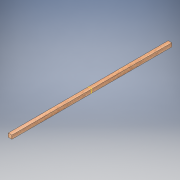
# Autodesk Inventor part: CAR_003_PoplarBrace
Saved by Autodesk Inventor 2018 (Build 220112000, 112)
## iProperties
Created: 2020-01-29
Part Number: CAR_003_PoplarBrace
Material: Wood (Birch)
Document SubType Name: Modeling
Designer: user
Mass: 41.2898 g
Surface Area: 240.193 cm^2
Volume: 75.0724 cm^3
Density: 0.55 g/cm^3
Appearance: Birch - Natural Polished
Author: user
Autodesk Inventor part; units mm, degrees
ref_plane "YZ Plane" through (0, 0, 0) normal (1, 0, 0) x (0, 1, 0)
ref_plane "XZ Plane" through (0, 0, 0) normal (0, 1, 0) x (-1, 0, 0)
ref_plane "XY Plane" through (0, 0, 0) normal (0, 0, 1) x (1, 0, 0)
sketch "Sketch1" plane through (0, 0, 0) normal (0, 0, 1) x (1, 0, 0)
  line L0 (0, 0) -> (12.7, 0)
  line L1 (12.7, 0) -> (12.7, 12.7)
  line L2 (12.7, 12.7) -> (0, 12.7)
  line L3 (0, 12.7) -> (0, 0)
  dimension "d0" = 12.7
  dimension "d1" = 12.7
  constraints: 8 end point, 2 parallel, 1 horizontal, 1 perpendicular
  measures "d0" distance of L2.end L1.end
  measures "d1" distance of L1.end L0.end
extrude "Extrusion1" add sketch "Sketch1" along normal mid plane 558.8
ref_plane "Work Plane2" through (0, 0, 0) normal (0, 0, 1) x (1, 0, 0)
sketch "Sketch2" plane through (0, 12.7, -279.4) normal (0, 1, 0) x (1, 0, 0)
  circle A0 centre (-130.048, -279.4) radius 273.05 construction
  line L0 (12.7, -558.8) -> (0, -558.8) projected
  line L1 (0, 0) -> (0, -558.8) projected
  circle A1 centre (-130.048, -279.4) radius 273.05
  circle A2 centre (-130.048, -279.4) radius 457.3654
  point P0 (0, -279.4)
  dimension "d4" = 546.1
  dimension "d5" = 279.4
  dimension "d6" = 130.048
  constraints: 3 centre point, 1 coincident, 1 concentric
  measures "d4" diameter of A0
  measures "d5" distance from line of L0 A0.centre
  measures "d6" distance from line of L1 A0.centre
body "Solid1"
